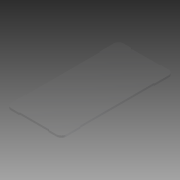
# Autodesk Inventor part: Macho Cristal_001
Saved by Autodesk Inventor 2015 (Build 190159000, 159)
## iProperties
Created: 2014-04-12
Part Number: Macho Cristal_001
Document SubType Name: Modeling
Designer: Oscar
Density: 1 g/cm^3
Material: Generic
Appearance: Clear - Light
Author: Oscar
Autodesk Inventor part; units mm, degrees
ref_plane "YZ Plane" through (0, 0, 0) normal (1, 0, 0) x (0, 1, 0)
ref_plane "XZ Plane" through (0, 0, 0) normal (0, 1, 0) x (-1, 0, 0)
ref_plane "XY Plane" through (0, 0, 0) normal (0, 0, 1) x (1, 0, 0)
sketch "Boceto1" plane through (0, 0, 0) normal (0, 0, 1) x (1, 0, 0)
  line L0 (-42.9, 87.4) -> (42.9, 87.4)
  line L1 (42.9, 87.4) -> (42.9, -87.4)
  line L2 (42.9, -87.4) -> (-42.9, -87.4)
  line L3 (-42.9, -87.4) -> (-42.9, 87.4)
  line L4 (42.9, 57.4) -> (41.8, 57.4)
  line L5 (41.8, 57.4) -> (41.8, -87.4)
  line L6 (-22.9, -87.4) -> (-22.9, -86.3)
  line L7 (-22.9, -86.3) -> (22.9, -86.3)
  line L8 (-42.9, -57.4) -> (-41.8, -57.4)
  line L9 (-41.8, -57.4) -> (-41.8, 95.5576)
  line L10 (-22.9, 87.4) -> (-22.9, 86.3)
  line L11 (-22.9, 86.3) -> (40.7099, 86.3)
  line L12 (26.8, 87.4) -> (-42.9, 87.4)
  line L13 (22.9, 87.4) -> (-22.9, 87.4)
  line L14 (-22.9, 87.4) -> (-22.9, 86.3)
  line L15 (-22.9, 86.3) -> (22.9, 86.3)
  line L16 (22.9, 86.3) -> (22.9, 87.4)
  line L17 (-42.9, 57.4) -> (-41.8, 57.4)
  line L18 (-41.8, 57.4) -> (-41.8, -57.4)
  line L19 (-41.8, -57.4) -> (-42.9, -57.4)
  line L20 (-42.9, -57.4) -> (-42.9, 57.4)
  line L21 (-22.9, -87.4) -> (22.9, -87.4)
  line L22 (22.9, -87.4) -> (22.9, -86.3)
  line L23 (22.9, -86.3) -> (-22.9, -86.3)
  line L24 (-22.9, -86.3) -> (-22.9, -87.4)
  line L25 (42.9, -57.4) -> (41.8, -57.4)
  line L26 (41.8, -57.4) -> (41.8, 57.4)
  line L27 (41.8, 57.4) -> (42.9, 57.4)
  line L28 (42.9, 57.4) -> (42.9, -57.4)
  point P0 (0, 0)
  point P1 (0, 87.4)
  point P2 (-42.9, 0)
  dimension "d0" = 85.8
  dimension "d1" = 174.8
  dimension "d18" = 30
  dimension "d19" = 30
  dimension "d21" = 20
  dimension "d22" = 30
  dimension "d25" = 20
  dimension "d26" = 20
  dimension "d27" = 30
  dimension "d28" = 20
  constraints: 58 end point, 13 parallel, 5 horizontal, 5 perpendicular, 5 point on line, 2 midpoint, 1 collinear, 1 horizontal alignment, 1 vertical alignment
  measures "d0" distance of L0.start L0.end
  measures "d1" distance of L2.end L0.start
  measures "d18" distance of L4.start L0.end
  measures "d19" distance of L25.start L1.end
  measures "d21" distance of L6.start L2.end
  measures "d22" distance of L8.start L2.end
  measures "d25" distance from line of L0.start L10
  measures "d26" distance from line of L0.end L16
  measures "d27" distance between parallel lines of L0 L17
  measures "d28" distance between parallel lines of L1 L22
extrude "Extrusión1" add sketch "Boceto1" along normal blind 3
extrude "Extrusión3" cut sketch "Boceto1" along normal up to surface (3 mm away) contours L0 L16 L11 L10 | L9 L8 L3 L17 | L1 L25 L5 L4 | L6 L7 L22 L2
fillet "Empalme2" radius 7.9 4 edges at (-42.9, 87.4, 1.5) (42.9, 87.4, 1.5) (42.9, -87.4, 1.5) (-42.9, -87.4, 1.5)
fillet "Empalme3" radius 0.5 16 edges at (-22.9, 87.4, 1.5) (-22.9, 86.3, 1.5) (22.9, 87.4, 1.5) (22.9, 86.3, 1.5) (42.9, 57.4, 1.5) (41.8, 57.4, 1.5) (42.9, -57.4, 1.5) (41.8, -57.4, 1.5) (22.9, -87.4, 1.5) (22.9, -86.3, 1.5) (-22.9, -87.4, 1.5) (-22.9, -86.3, 1.5) (-42.9, -57.4, 1.5) (-41.8, -57.4, 1.5) (-42.9, 57.4, 1.5) (-41.8, 57.4, 1.5)
body "Solid1"
